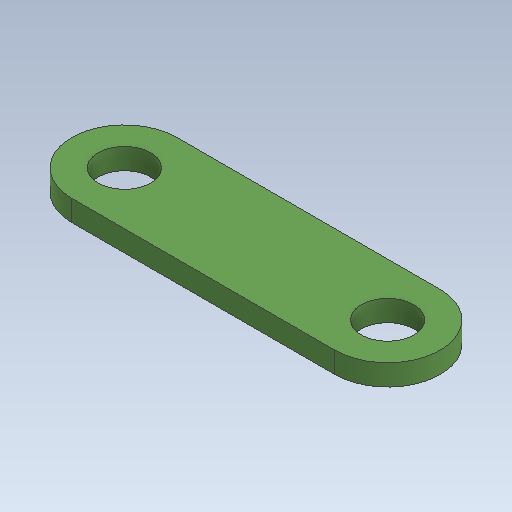
# Autodesk Inventor part: Input
Saved by Autodesk Inventor 2020.1 (Build 241239000, 239)
## iProperties
Created: 2019-08-08
Part Number: Input
Material: Generic
Document SubType Name: Modeling
Designer: sshel
Density: 1 g/cm^3
Appearance: Default
Mass: 9480.57 g
Surface Area: 5188.4 cm^2
Volume: 9480.57 cm^3
Author: sshel
Autodesk Inventor part; units mm, degrees
ref_plane "YZ Plane" through (0, 0, 0) normal (1, 0, 0) x (0, 1, 0)
ref_plane "XZ Plane" through (0, 0, 0) normal (0, 1, 0) x (-1, 0, 0)
ref_plane "XY Plane" through (0, 0, 0) normal (0, 0, 1) x (1, 0, 0)
sketch "Sketch1" plane through (0, 0, 0) normal (0, 1, 0) x (-1, 0, 0)
  line L0 (-317.5, 127) -> (317.5, 127)
  line L1 (317.5, 127) -> (317.5, -127) construction
  line L2 (317.5, -127) -> (-317.5, -127)
  line L3 (-317.5, -127) -> (-317.5, 127) construction
  line L4 (-317.5, 127) -> (317.5, -127) construction
  line L5 (317.5, 127) -> (-317.5, -127) construction
  arc A0 (317.5, -127) -> (317.5, 127) centre (317.5, 0) ccw
  arc A1 (-317.5, 127) -> (-317.5, -127) centre (-317.5, 0) ccw
  circle A2 centre (317.5, 0) radius 63.5
  circle A3 centre (-317.5, 0) radius 63.5
  point P0 (0, 0)
  dimension "d0" = 635
  dimension "d1" = 254
  dimension "d2" = 127
  dimension "d3" = 127
  constraints: 12 end point, 4 centre point, 4 point on circle, 4 tangent, 2 coincident, 2 midpoint, 2 parallel, 1 horizontal, 1 perpendicular
  measures "d0" distance of L1.end L2.end
  measures "d1" distance of L2.end L0.start
  measures "d2" diameter of A2
  measures "d3" diameter of A3
extrude "Extrusion1" add sketch "Sketch1" along normal blind 50.8
body "Solid1"
